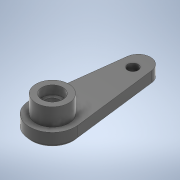
# Autodesk Inventor part: RCT-P070_servo_linkage
Saved by Autodesk Inventor 2020 (Build 240168000, 168)
## iProperties
Created: 2019-12-03
Part Number: RCT-P070_servo_linkage
Material: Generic
Document SubType Name: Modeling
Designer: maste
Density: 1 g/cm^3
Appearance: Smooth - Black
Author: maste
Autodesk Inventor part; units mm, degrees
ref_plane "YZ Plane" through (0, 0, 0) normal (1, 0, 0) x (0, 1, 0)
ref_plane "XZ Plane" through (0, 0, 0) normal (0, 1, 0) x (-1, 0, 0)
ref_plane "XY Plane" through (0, 0, 0) normal (0, 0, 1) x (1, 0, 0)
sketch "Sketch1" plane through (0, 0, 0) normal (0, 1, 0) x (-1, 0, 0)
  arc A0 (6.4507, -0.7992) -> (-6.4507, -0.7992) centre (0, 0) ccw
  arc A1 (-3.4734, -24.8303) -> (3.4734, -24.8303) centre (0, -24.4) ccw
  line L0 (0, -34.78) -> (0, 13.38) projected
  line L1 (6.4507, -0.7992) -> (3.4734, -24.8303)
  line L2 (-6.4507, -0.7992) -> (-3.4734, -24.8303)
  circle A2 centre (0, -22.9) radius 1.5
  dimension "d0" = 13
  dimension "d1" = 7
  dimension "d2" = 34.4
  dimension "d3" = 3
  dimension "d4" = 1.5
  constraints: 4 end point, 4 point on circle, 4 tangent, 3 centre point, 2 point on line, 1 coincident
  measures "d0" diameter of A0
  measures "d1" diameter of A1
  measures "d3" diameter of A2
  measures "d4" distance of A1.centre A2.centre
extrude "Extrusion1" add sketch "Sketch1" along normal blind 3 contours L1 A1 L0 A2 A0 | L0 A2 A1 L2 A0
sketch "Sketch2" plane through (0, 3, 0) normal (0, 1, 0) x (1, 0, 0)
  circle A0 centre (0, 0) radius 4.675
  dimension "d7" = 9.35
  constraints: 1 centre point, 1 coincident
  measures "d7" diameter of A0
extrude "Extrusion2" add sketch "Sketch2" along normal blind 5
sketch "Sketch3" plane through (0, 8, 0) normal (0, 1, 0) x (1, 0, 0)
  circle A0 centre (0, 0) radius 3
  dimension "d10" = 6
  constraints: 1 centre point, 1 coincident
  measures "d10" diameter of A0
extrude "Extrusion3" cut sketch "Sketch3" against normal blind 2.5
sketch "Sketch4" plane through (0, 0, 0) normal (0, -1, 0) x (1, 0, 0)
  circle A0 centre (0, 0) radius 6
  dimension "d13" = 12
  constraints: 1 centre point, 1 coincident
  measures "d13" diameter of A0
extrude "Extrusion4" add sketch "Sketch4" along normal blind 1
fillet "Fillet1" radius 0.5 1 edges at (-6, -1, 0)
sketch "Sketch5" plane through (0, -1, 0) normal (0, -1, 0) x (1, 0, 0)
  circle A0 centre (0, 0) radius 3
  dimension "d17" = 6
  constraints: 1 centre point, 1 coincident
  measures "d17" diameter of A0
extrude "Extrusion5" cut sketch "Sketch5" against normal blind 4
sketch "Sketch6" plane through (0, 3, 0) normal (0, -1, 0) x (1, 0, 0)
  circle A0 centre (0, 0) radius 2
  dimension "d20" = 4
  constraints: 1 centre point, 1 coincident
  measures "d20" diameter of A0
extrude "Extrusion6" cut sketch "Sketch6" against normal through all
body "Solid1"
